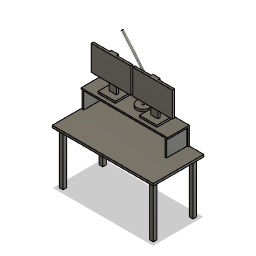
kataszgpolc v2 (Autodesk Fusion 360 design; units mm, degrees)
Autodesk Fusion 360 part; units mm, degrees
sketch "Sketch1" plane through (0, 0, 0) normal (0, 1, 0) x (1, 0, 0)
  line L0 (600, -150) -> (-600, -150)
  line L1 (-600, -150) -> (-600, 150)
  line L2 (-600, 150) -> (600, 150)
  line L3 (600, 150) -> (600, -150)
  line L4 (600, -150) -> (-600, 150) construction
  line L5 (-600, -150) -> (600, 150) construction
  line L6 (-575, 225) -> (-575, -250) construction
  line L7 (-565, 150) -> (-585, 150)
  line L8 (-585, 150) -> (-585, -150)
  line L9 (-585, -150) -> (-565, -150)
  line L10 (-565, -150) -> (-565, 150)
  line L11 (-565, 150) -> (-585, -150) construction
  line L12 (-585, 150) -> (-565, -150) construction
  line L13 (0, 150) -> (0, -150) construction
  line L14 (565, 150) -> (585, 150)
  line L15 (565, -150) -> (565, 150)
  line L16 (585, 150) -> (585, -150)
  line L17 (585, -150) -> (565, -150)
  line L18 (-600, 150) -> (600, 150)
  line L19 (600, 150) -> (600, 130)
  line L20 (600, 130) -> (-600, 130)
  line L21 (-600, 130) -> (-600, 150)
  point P0 (-575, 0)
  dimension "d1" = 1200
  dimension "d2" = 300
  dimension "d3" = 25
  dimension "d4" = 20
  dimension "d5" = 20
  constraint horizontal L0
  constraint perpendicular L0 L1
  constraint parallel L0 L2
  constraint parallel L1 L3
  constraint coincident L4 origin
  constraint coincident L5 origin
  constraint perpendicular L2 L6
  constraint horizontal L7
  constraint perpendicular L7 L8
  constraint parallel L7 L9
  constraint parallel L8 L10
  constraint coincident L11 P0
  constraint coincident L12 P0
  constraint coincident L6 P0
  constraint midpoint L2 L13.start
  constraint midpoint L0 L13.end
  constraint symmetric L7.start L13 L14.start
  constraint symmetric L7.end L13 L14.end
  constraint symmetric L8.end L13 L16.end
  constraint symmetric L9.end L13 L15.start
  constraint horizontal L18
  constraint vertical L19
  constraint horizontal L20
  constraint vertical L21
  measures "d1" distance of L1.end L2.end
  measures "d2" distance of L0.end L1.end
  measures "d3" distance of L1 L6
  measures "d4" distance of L8.end L9.end
  measures "d5" distance of L1.end L20.end
extrude "Extrude1" add sketch "Sketch1" along normal blind 20 makes body 1
extrude "Extrude2" add sketch "Sketch1" against normal blind 230 contours L0 L15 L16 L17 L20 | L2 L3 L16 L18 L19 L20 | L2 L14 L15 L16 L18 L20 | L0 L8 L9 L10 L20 | L2 L10 L15 L18 L20 | L2 L7 L8 L10 L18 L20 | L1 L2 L8 L18 L20 L21 bodies 1
copy_body "Body->Comp5" bodies 1 removing the originals makes body 2 in component "polc"
sketch "Sketch2" plane through (0, 0, 0) normal (0, 0, 1) x (1, 0, 0)
  line L0 (-471.3089, 484.3861) -> (78.6911, 484.3861)
  line L1 (78.6911, 484.3861) -> (78.6911, 134.3861)
  line L2 (78.6911, 134.3861) -> (-471.3089, 134.3861)
  line L3 (-471.3089, 134.3861) -> (-471.3089, 484.3861)
  dimension "d10" = 550
  dimension "d11" = 350
  constraint horizontal L0
  constraint vertical L1
  constraint horizontal L2
  constraint vertical L3
  measures "d10" distance of L0.start L0.end
  measures "d11" distance of L0.start L2.end
extrude "Extrude3" add sketch "Sketch2" along normal blind 30 separate body makes body 3
ref_plane "WorkPlane1" through (-196.3089, 484.3861, 15) normal (0, 1, 0) x (-1, 0, 0)
sketch "Sketch3" plane through (-196.3089, 484.3861, 15) normal (0, 1, 0) x (1, 0, 0)
  line L0 (-50, 50) -> (50, 50)
  line L1 (50, 50) -> (50, 20)
  line L2 (50, 20) -> (-50, 20)
  line L3 (-50, 20) -> (-50, 50)
  constraint horizontal L0
  constraint vertical L1
  constraint horizontal L2
  constraint vertical L3
extrude "Extrude4" add sketch "Sketch3" against normal blind 470 separate body makes body 4
ref_plane "WorkPlane2" through (-196.3089, 14.3861, -20) normal (0, -1, 0) x (0, 0, -1)
sketch "Sketch4" plane through (-196.3089, 14.3861, -20) normal (0, -1, 0) x (1, 0, 0)
  line L0 (120, -100) -> (-120, -100)
  line L1 (-120, -100) -> (-120, 100)
  line L2 (-120, 100) -> (120, 100)
  line L3 (120, 100) -> (120, -100)
  line L4 (120, -100) -> (-120, 100) construction
  line L5 (-120, -100) -> (120, 100) construction
  dimension "d18" = 240
  dimension "d19" = 200
  constraint horizontal L0
  constraint perpendicular L0 L1
  constraint parallel L0 L2
  constraint parallel L1 L3
  constraint coincident L4 origin
  constraint coincident L5 origin
  measures "d18" distance of L1.end L2.end
  measures "d19" distance of L0.end L1.end
extrude "Extrude5" add sketch "Sketch4" along normal blind 25 bodies 4
move_body "Move1" bodies 4 to x (1, 0, 0) y (0, 1, 0) z (0, 0, 1) at (0, 0, 10)
combine "Combine1" operation add target body 3 tool bodies 4
move_body "Move2" bodies 3 to x (1, 0, 0) y (0, 1, 0) z (0, 0, 1) at (0, 100, 0)
copy_body "CopyPasteBodies1" bodies 3 makes body 5
move_body "Move3" bodies 5 to x (1, 0, 0) y (0, 1, 0) z (0, 0, 1) at (575, 0, 0)
move_body "Move4" bodies 3 5 to x (1, 0, 0) y (0, 1, 0) z (0, 0, 1) at (-100, 0, 0)
move_body "Move5" bodies 3 5 to x (1, 0, 0) y (0, 1, 0) z (0, 0, 1) at (176.3089, -69.3861, -90)
move_body "Move6" bodies 3 5 to x (1, 0, 0) y (0, 1, 0) z (0, 0, 1) at (-175, 0, 100)
ref_plane "WorkPlane3" through (0, -230, 0) normal (0, -1, 0) x (0, 0, -1)
copy_body "Body->Comp6" bodies 3 removing the originals makes body 6 in component "monitor"
copy_body "Body->Comp7" bodies 5 removing the originals makes body 7 in component "monitor (1)"
sketch "Sketch5" plane through (0, -230, 0) normal (0, -1, 0) x (1, 0, 0)
  line L0 (700, 350) -> (-700, 350)
  line L1 (-700, 350) -> (-700, -350)
  line L2 (-700, -350) -> (700, -350)
  line L3 (700, -350) -> (700, 350)
  line L4 (700, 350) -> (-700, -350) construction
  line L5 (-700, 350) -> (700, -350) construction
  dimension "d23" = 700
  constraint horizontal L0
  constraint perpendicular L0 L1
  constraint parallel L0 L2
  constraint parallel L1 L3
  constraint coincident L4 origin
  constraint coincident L5 origin
  measures "d23" distance of L0.end L1.end
extrude "Extrude6" add sketch "Sketch5" along normal blind 30 separate body makes body 8
sketch "Sketch6" plane through (0, -260, 0) normal (0, -1, 0) x (1, 0, 0)
  line L0 (700, -350) -> (700, 350)
  line L1 (700, 350) -> (-700, 350)
  line L2 (-700, 350) -> (-700, -350)
  line L3 (-700, -350) -> (700, -350)
  line L4 (-650, 300) -> (-600, 300)
  line L5 (-600, 300) -> (-600, 250)
  line L6 (-600, 250) -> (-650, 250)
  line L7 (-650, 250) -> (-650, 300)
  line L8 (0, 1.75) -> (0, 22.5)
  line L9 (600, 300) -> (600, 250)
  line L10 (600, 250) -> (650, 250)
  line L11 (650, 250) -> (650, 300)
  line L12 (650, 300) -> (600, 300)
  line L13 (1.75, 0) -> (22.5, 0)
  line L14 (-600, -300) -> (-600, -250)
  line L15 (-650, -300) -> (-600, -300)
  line L16 (-600, -250) -> (-650, -250)
  line L17 (-650, -250) -> (-650, -300)
  line L18 (600, -300) -> (600, -250)
  line L19 (650, -300) -> (600, -300)
  line L20 (650, -250) -> (650, -300)
  line L21 (600, -250) -> (650, -250)
  dimension "d26" = 50
  dimension "d27" = 50
  constraint horizontal L4
  constraint vertical L5
  constraint horizontal L6
  constraint vertical L7
  constraint symmetric L4.start L8 L11.end
  constraint symmetric L4.end L8 L9.start
  constraint symmetric L5.end L8 L9.end
  constraint symmetric L6.end L8 L10.end
  constraint symmetric L4.start L13 L15.start
  constraint symmetric L4.end L13 L14.start
  constraint symmetric L5.end L13 L14.end
  constraint symmetric L6.end L13 L16.end
  constraint symmetric L9.start L13 L18.start
  constraint symmetric L9.end L13 L18.end
  constraint symmetric L10.end L13 L20.start
  constraint symmetric L11.end L13 L19.start
  measures "d26" distance of L2 L7
  measures "d27" distance of L1 L4
extrude "Extrude7" add sketch "Sketch6" along normal blind 720 contours L4 L5 L6 L7 | L9 L10 L11 L12 | L14 L15 L16 L17 | L18 L19 L20 L21 bodies 8
move_body "Move7" bodies 8 to x (1, 0, 0) y (0, 1, 0) z (0, 0, 1) at (0, 0, 200)
copy_body "Body->Comp8" bodies 8 removing the originals makes body 9 in component "asztal"
ref_plane "WorkPlane4" through (0, -230, 200) normal (0, 1, 0) x (-1, 0, 0)
sketch "Sketch7" plane through (0, -230, 200) normal (0, 1, 0) x (1, 0, 0)
  circle A0 centre (650, -250) radius 90
  dimension "d31" = 180
  measures "d31" diameter of A0
extrude "Extrude1'" add sketch "Sketch7" along normal blind 30 separate body makes body 10 in component "asztal"
sketch "Sketch8" plane through (0, -200, 0) normal (0, 1, 0) x (-1, 0, 0)
  circle A0 centre (-650, 450) radius 90
  circle A1 centre (-650, 450) radius 15
  dimension "d34" = 30
  constraint concentric A0 A1
  measures "d34" diameter of A1
extrude "Extrude2'" add sketch "Sketch8" along normal blind 400 contours A1 bodies 9 10 in component "asztal"
sketch "Sketch9" plane through (0, 200, 0) normal (0, 1, 0) x (-1, 0, 0)
  circle A0 centre (-650, 450) radius 15
  circle A1 through (-635, 449.9942, 0.016) (-657.5, 459.9454, 8.3661) (-657.5, 440.043, -8.334)
  line L0 (-635, 449.9751) -> (-665, 449.9751) construction
extrude "Extrude4'" add sketch "Sketch9" against normal blind 200 contours A1 in plane through (0, -21.5695, 185.9189) normal (0, 0.766044, -0.642788) bodies 10 in component "asztal"
extrude "Extrude3'" add sketch "Sketch9" along normal blind 450 contours A1 in plane through (0, -21.5695, 185.9189) normal (0, 0.766044, -0.642788) bodies 10 in component "asztal"
copy_body "CutPasteBodies2" bodies 10 removing the originals makes body 11
copy_body "Body->Comp9" bodies 11 removing the originals makes body 12 in component "Component"
move_body "Move1'" bodies 12 to x (1, 0, 0) y (0, 1, 0) z (0, 0, 1) at (-650, 250, -450) in component "Component"
component "polc" placed x (1, 0, 0) y (0, 1, 0) z (0, 0, 1) at (0, 0, 0)
component "monitor" placed x (1, 0, 0) y (0, 1, 0) z (0, 0, 1) at (0, 0, 0)
component "monitor (1)" placed x (1, 0, 0) y (0, 1, 0) z (0, 0, 1) at (0, 0, 0)
component "asztal" placed x (1, 0, 0) y (0, 1, 0) z (0, 0, 1) at (0, 0, 0)
component "Component" placed x (1, 0, 0) y (0, 1, 0) z (0, 0, 1) at (0, 0, 0)
named bodies: "polc", "monitor", "monitor (1)", "asztal"
